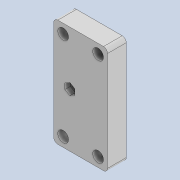
# Autodesk Inventor part: 10_Mountinplate_Mirrors_v0
Saved by Autodesk Inventor 2022 (Build 260153000, 153)
## iProperties
Created: 2022-05-18
Part Number: 10_Mountinplate_Mirrors_v0
Material: Generisch
Document SubType Name: Modeling
Designer: diederichbenedict
Density: 1 g/cm^3
Appearance: Vorgabe
Author: diederichbenedict
Autodesk Inventor part; units mm, degrees
ref_plane "YZ Plane" through (0, 0, 0) normal (1, 0, 0) x (0, 1, 0)
ref_plane "XZ Plane" through (0, 0, 0) normal (0, 1, 0) x (-1, 0, 0)
ref_plane "XY Plane" through (0, 0, 0) normal (0, 0, 1) x (1, 0, 0)
ref_plane "Arbeitsebene1" through (0.0075, -0.0423, 0) normal (0, 0, 1) x (1, 0, 0)
sketch "Skizze1" plane through (0.0075, -0.0423, 0) normal (0, 0, 1) x (1, 0, 0)
  line L0 (0.635, 25.527) -> (10.16, 25.527) projected
  line L1 (0.635, 25.527) -> (0.635, 0) projected
  line L2 (0.635, 0) -> (10.16, 0) projected
  line L3 (10.16, 0) -> (10.16, 25.527) projected
  line L4 (30.08, -27.3) -> (-3.92, -27.3)
  line L5 (-6.92, -24.3) -> (-6.92, 49.7)
  line L6 (-3.92, 52.7) -> (30.08, 52.7)
  line L7 (33.08, -27.3) -> (-6.92, 52.7) construction
  line L8 (-6.92, -27.3) -> (33.08, 52.7) construction
  arc A0 (30.08, -27.3) -> (33.08, -24.3) centre (30.08, -24.3) ccw
  arc A1 (-6.92, -24.3) -> (-3.92, -27.3) centre (-3.92, -24.3) ccw
  arc A2 (-3.92, 52.7) -> (-6.92, 49.7) centre (-3.92, 49.7) ccw
  arc A3 (33.08, 49.7) -> (30.08, 52.7) centre (30.08, 49.7) ccw
  circle A4 centre (5.08, 12.7) radius 2.3813
  line L9 (33.08, -24.3) -> (33.08, 49.7)
  point P0 (-0.0075, 0.0423)
  point P1 (13.08, 12.7)
  dimension "d1" = 80
  dimension "d2" = 3
  dimension "d7" = 0
  dimension "d8" = 8
  constraints: 12 end point, 8 point on circle, 7 tangent, 6 point on line, 5 centre point, 3 equal radius, 1 horizontal, 1 midpoint, 1 parallel, 1 perpendicular, 1 vertical, 2 other
  measures "d1" distance of L8.start L7.end
  measures "d2" radius of A0
  measures "d7" vertical distance of A4.centre point (13.08, 12.7)
  measures "d8" distance of point (13.08, 12.7) A4.centre
ref_plane "Arbeitsebene2" through (291.5074, -13.3966, 8.6065) normal (0, 0, 1) x (0.898794, -0.4383711, 0)
extrude "Extrusion1" add sketch "Skizze1" along normal blind 12.612 contours L0 L3 L2 L1 | L4 A1 L5 A2 L6 A3 L9 A0
sketch "Skizze3" plane through (0.0075, -0.0423, 0) normal (0, 0, -1) x (-1, 0, 0)
  arc A0 (-30.08, 52.7) -> (-33.08, 49.7) centre (-30.08, 49.7) ccw projected
  line L0 (-33.08, -24.3) -> (-33.08, 49.7) projected
  arc A1 (-33.08, -24.3) -> (-30.08, -27.3) centre (-30.08, -24.3) ccw projected
  line L1 (3.92, -27.3) -> (-30.08, -27.3) projected
  arc A2 (3.92, -27.3) -> (6.92, -24.3) centre (3.92, -24.3) ccw projected
  line L2 (6.92, 49.7) -> (6.92, -24.3) projected
  arc A3 (6.92, 49.7) -> (3.92, 52.7) centre (3.92, 49.7) ccw projected
  line L3 (-30.08, 52.7) -> (3.92, 52.7) projected
  circle A4 centre (-5.08, 12.7) radius 2.3813 projected
  line L4 (-26.08, 45.7) -> (-0.08, 45.7)
  line L5 (-0.08, 45.7) -> (-0.08, -20.3)
  line L6 (-0.08, -20.3) -> (-26.08, -20.3)
  line L7 (-26.08, -20.3) -> (-26.08, 45.7)
  point P0 (0.0075, 0.0423)
  dimension "d9" = 7
  constraints: 8 end point, 3 other
  measures "d9" distance between parallel lines of L0 L7
hole "Bohrung1" at (26.0875, 45.6577, 0) at (26.0875, -20.3423, 0) at (0.0875, -20.3423, 0) at (0.0875, 45.6577, 0) direction (0, 0, 1) diameter 8 depth 15 tip angle 118
sketch "Skizze4" plane through (-6.9125, -24.3423, 0) normal (-1, 0, 0) x (0, 0, 1)
  circle A0 centre (-6.731, 17.9923) radius 7.366 projected
  circle A1 centre (-6.731, 17.9923) radius 9.366
  circle A2 centre (-6.731, 56.05) radius 7.366
  circle A3 centre (-6.731, 56.05) radius 9.366
  point P0 (0, 24.3423)
  dimension "d17" = 2
  constraints: 3 centre point, 1 equal radius, 2 other
  measures "d17" radial gap between concentric circles of A0 A1
ref_plane "Arbeitsebene3" through (0, -11.176, -49.276) normal (-1, 0, 0) x (0, 0.0000004, 1)
extrude "Extrusion2" cut sketch "Skizze4" against normal up to surface (6.9125 mm away) contours A0 | A1 | A2 | A3
sketch "Skizze5" plane through (0.0075, -0.0423, 0) normal (0, 0, -1) x (-1, 0, 0)
  circle A0 centre (-5.08, 12.7) radius 2.3813 projected
  line L0 (6.92, -12.8204) -> (0.0075, -12.8204) projected
  line L1 (0.0075, -12.8204) -> (0.0075, 0.2051) projected
  line L2 (0.0075, 0.2051) -> (6.92, 0.2051) projected
  line L3 (6.92, 49.7) -> (6.92, 38.2627) projected
  arc A1 (6.92, 49.7) -> (3.92, 52.7) centre (3.92, 49.7) ccw projected
  line L4 (-30.08, 52.7) -> (3.92, 52.7) projected
  arc A2 (-30.08, 52.7) -> (-33.08, 49.7) centre (-30.08, 49.7) ccw projected
  line L5 (-33.08, -24.3) -> (-33.08, 49.7) projected
  arc A3 (-33.08, -24.3) -> (-30.08, -27.3) centre (-30.08, -24.3) ccw projected
  line L6 (3.92, -27.3) -> (-30.08, -27.3) projected
  arc A4 (3.92, -27.3) -> (6.92, -24.3) centre (3.92, -24.3) ccw projected
  line L7 (6.92, -12.8204) -> (6.92, -24.3) projected
  circle A5 centre (-0.08, 45.7) radius 4 projected
  circle A6 centre (-26.08, -20.3) radius 4 projected
  circle A7 centre (-26.08, 45.7) radius 4 projected
  circle A8 centre (-0.08, -20.3) radius 4 projected
  line L8 (-0.6275, 29.1761) -> (-10.1525, 29.1761) projected
  line L9 (-0.6275, -2.2391) -> (-10.1525, -2.2391) projected
  line L10 (-10.1525, -2.2391) -> (-10.1525, 29.1761)
  line L11 (-0.6275, 29.1761) -> (-0.6275, -2.2391)
  line L12 (0.0075, 0.2051) -> (0.0075, -12.8204) projected
  line L13 (-10.3525, 29.3761) -> (-0.4275, 29.3761)
  line L14 (-0.4275, 29.3761) -> (-0.4275, -2.4391)
  line L15 (-0.4275, -2.4391) -> (-10.3525, -2.4391)
  line L16 (-10.3525, -2.4391) -> (-10.3525, 29.3761)
  line L17 (6.92, 25.2373) -> (6.92, 0.2051) projected
  line L18 (6.92, 25.2373) -> (0.0075, 25.2373) projected
  line L19 (0.0075, 25.2373) -> (0.0075, 38.2627) projected
  line L20 (0.0075, 38.2627) -> (6.92, 38.2627) projected
  line L21 (-12.6873, 36.83) -> (-19.1643, 36.83)
  line L22 (-12.6873, -11.811) -> (-19.1643, -11.811)
  line L23 (-12.6873, 17.399) -> (-12.6873, 4.5974)
  line L24 (-19.7993, 21.1275) -> (-19.7993, 26.543)
  line L25 (-12.6873, -11.811) -> (-19.7993, -11.811)
  line L26 (-19.7993, -11.811) -> (-19.7993, 36.83)
  line L27 (-19.7993, 36.83) -> (-12.6873, 36.83)
  line L28 (-12.6873, 36.83) -> (-12.6873, -11.811)
  line L29 (-19.9993, 37.03) -> (-19.9993, -12.011)
  line L30 (-19.9993, -12.011) -> (-12.4873, -12.011)
  line L31 (-12.4873, -12.011) -> (-12.4873, 37.03)
  line L32 (-12.4873, 37.03) -> (-19.9993, 37.03)
  line L33 (-19.9993, -12.011) -> (-22.9993, -12.011)
  line L34 (-22.9993, -12.011) -> (-22.9993, 37.03)
  line L35 (-22.9993, 37.03) -> (-19.9993, 37.03)
  line L36 (-19.9993, 37.03) -> (-19.9993, -12.011)
  line L37 (0, -0.127) -> (0, 25.4)
  line L38 (0, -0.127) -> (0, 25.4)
  line L39 (-0.4275, -2.4391) -> (0.0075, -2.4391)
  line L40 (0.2725, 0.2051) -> (0.2725, 25.2373)
  line L41 (0.2725, 29.3761) -> (-0.4275, 29.3761)
  line L42 (-0.4275, 29.3761) -> (-0.4275, -2.4391)
  point P0 (0.0075, 0.0423)
  point P1 (-19.9993, 37.03)
  point P2 (0.0075, 29.3761)
  dimension "d20" = 0.2
  dimension "d26" = 0.2
  dimension "d27" = 3
  dimension "d28" = 0.7
  constraints: 56 end point, 9 parallel, 5 horizontal, 5 vertical, 4 perpendicular, 3 point on line, 16 other
  measures "d20" distance between parallel lines of L11 L14
  measures "d26" distance between parallel lines of L26 L29
  measures "d27" distance of L34.end L35.end
  measures "d28" distance of L41.end L41.start
ref_plane "Arbeitsebene4" through (-0.1034, 27.5049, -1.27) normal (0, 0.0000004, 1) x (1, 0, 0)
extrude "Extrusion3" add sketch "Skizze5" along normal up to surface (1.27 mm away) contours L7 A4 L6 A3 L5 A2 L4 A1 L3 L20 L19 L41 L13 L16 L15 L39 L1 L0 | L40 L18 L17 L2
sketch "Sketch6" plane through (0.0075, -0.0423, 12.612) normal (0, 0, 1) x (1, 0, 0)
  circle A0 centre (5.08, 12.7) radius 2.3813 projected
  line L0 (8.8085, 14.7861) -> (8.7509, 10.5141)
  line L1 (8.7509, 10.5141) -> (5.0224, 8.428)
  line L2 (5.0224, 8.428) -> (1.3515, 10.6139)
  line L3 (1.3515, 10.6139) -> (1.4091, 14.8859)
  line L4 (1.4091, 14.8859) -> (5.1376, 16.972)
  line L5 (5.1376, 16.972) -> (8.8085, 14.7861)
  point P0 (-0.0075, 0.0423)
  dimension "d23" = 3.7
  constraints: 12 end point, 1 coincident, 13 other
  measures "d23" distance from line of L4 A0.centre
extrude "Extrusion4" cut sketch "Sketch6" against normal blind 4 contours A0 | L0 L1 L2 L3 L4 L5
fillet "Fillet1" radius 0.5 8 edges at (-0.265, 12.6788, -1.27) (5.18, -2.4814, -1.27) (10.36, 13.4262, -1.27) (5.18, 29.3338, -1.27) (23.0068, 12.4672, -1.27) (12.4948, 12.4672, -1.27) (17.7508, 36.9877, -1.27) (17.7508, -12.0533, -1.27)
